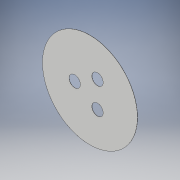
# Autodesk Inventor part: 부품1
Saved by Autodesk Inventor 2019 (Build 230136000, 136)
## iProperties
Created: 2019-08-28
Part Number: 부품1
Material: 일반
Document SubType Name: Sheet Metal
Designer: khopa
Density: 1 g/cm^3
Sheet Metal Rule: 기본값_mm
Appearance: 기본값
Author: khopa
Autodesk Inventor part; units mm, degrees
ref_plane "YZ Plane" through (0, 0, 0) normal (1, 0, 0) x (0, 1, 0)
ref_plane "XZ Plane" through (0, 0, 0) normal (0, 1, 0) x (-1, 0, 0)
ref_plane "XY Plane" through (0, 0, 0) normal (0, 0, 1) x (1, 0, 0)
sketch "스케치1" plane through (0, 0, 0) normal (0, 0, 1) x (1, 0, 0)
  circle A0 centre (0, 0) radius 125
  dimension "d0" = 250
  measures "d0" diameter of A0
extrude "판1" add sketch "스케치1" along normal blind 0.5
sketch "스케치2" plane through (0, 0, 0.5) normal (0, 0, 1) x (1, 0, 0)
  circle A0 centre (-40, 0) radius 15
  point P0 (0, 0)
  dimension "d2" = 30
  dimension "d4" = 40
  constraints: 1 centre point
  measures "d2" diameter of A0
  measures "d4" distance of point (0, 0) A0.centre
extrude "돌출1" cut sketch "스케치2" against normal blind 10
pattern_circular "원형 패턴1" count 3 over 360 about axis through (0, 0, 0) along (0, 0, 1) of "돌출1"
equation "\"TransitionRadius\" = BendRadius"
equation "\"BendRadius\" = 0.5"
